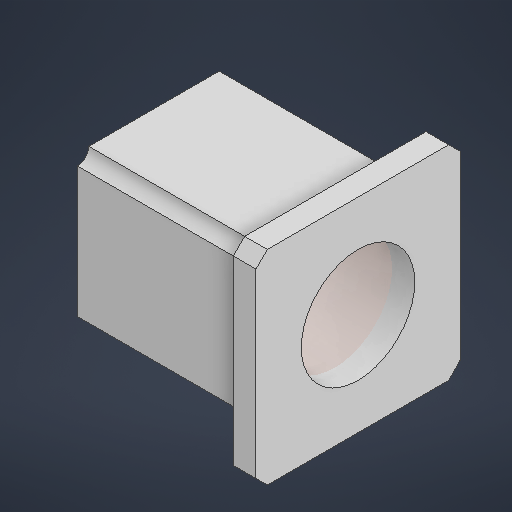
# Autodesk Inventor part: переходник
Saved by Autodesk Inventor 2026 (Build 300175000, 175)
## iProperties
Created: 2025-08-21
Part Number: переходник
Material: Типовые
Document SubType Name: Modeling
Designer: danil
Density: 1 g/cm^3
Appearance: По умолчанию
Author: danil
Autodesk Inventor part; units mm, degrees
ref_plane "YZ Plane" through (0, 0, 0) normal (1, 0, 0) x (0, 1, 0)
ref_plane "XZ Plane" through (0, 0, 0) normal (0, 1, 0) x (-1, 0, 0)
ref_plane "XY Plane" through (0, 0, 0) normal (0, 0, 1) x (1, 0, 0)
sketch "Эскиз1" plane through (0, 0, 0) normal (1, 0, 0) x (0, 1, 0)
  line L0 (6.75, 6.75) -> (-6.75, 6.75)
  line L1 (-6.75, 6.75) -> (-6.75, -6.75)
  line L2 (-6.75, -6.75) -> (6.75, -6.75)
  line L3 (6.75, -6.75) -> (6.75, 6.75)
  circle A0 centre (0, 0) radius 5
  dimension "d0" = 13.5
  dimension "d1" = 13.5
  dimension "d2" = 6.75
  dimension "d3" = 6.75
  dimension "d4" = 10
  constraints: 8 end point, 2 parallel, 1 centre point, 1 coincident, 1 horizontal, 1 perpendicular
  measures "d0" distance of L1.end L2.end
  measures "d1" distance of L2.end L0.start
  measures "d2" horizontal distance of point (0, 0) L2.end
  measures "d3" horizontal distance of point (0, 0) L2.end
  measures "d4" diameter of A0
extrude "Выдавливание1" add sketch "Эскиз1" along normal blind 16
ref_plane "РабПлоскость1" through (16, 0, 0) normal (1, 0, 0) x (0, 0, -1)
sketch "Эскиз2" plane through (16, 0, 0) normal (1, 0, 0) x (0, 0, -1)
  line L0 (6.75, -6.75) -> (6.75, 6.75) projected
  circle A0 centre (6.75, 6.75) radius 1
  line L1 (6.75, 6.75) -> (-6.75, 6.75) projected
  circle A1 centre (-6.75, 6.75) radius 1
  line L2 (-6.75, -6.75) -> (6.75, -6.75) projected
  circle A2 centre (-6.75, -6.75) radius 1
  circle A3 centre (6.75, -6.75) radius 1
  point P0 (0, 0)
  dimension "d8" = 2
  dimension "d9" = 2
  dimension "d10" = 2
  dimension "d11" = 2
  constraints: 4 centre point, 1 coincident
  measures "d8" diameter of A0
  measures "d9" diameter of A3
  measures "d10" diameter of A2
  measures "d11" diameter of A1
extrude "Выдавливание2" cut sketch "Эскиз2" against normal blind 16
sketch "Эскиз3" plane through (16, 0, 0) normal (1, 0, 0) x (0, 0, -1)
  line L0 (-9, -9) -> (9, -9)
  line L1 (9, -9) -> (9, 9)
  line L2 (9, 9) -> (-9, 9)
  line L3 (-9, 9) -> (-9, -9)
  line L4 (-9, -9) -> (9, 9) construction
  line L5 (9, -9) -> (-9, 9) construction
  circle A0 centre (0, 0) radius 5
  dimension "d14" = 18
  dimension "d15" = 18
  constraints: 12 end point, 2 midpoint, 2 parallel, 1 centre point, 1 coincident, 1 horizontal, 1 perpendicular
  measures "d14" distance of L1.end L2.end
  measures "d15" distance of L0.end L1.end
extrude "Выдавливание3" add sketch "Эскиз3" along normal blind 2
chamfer "Фаска1" distance 1 angle 45 4 edges at (17, 9, 9) (17, 9, -9) (17, -9, 9) (17, -9, -9)
